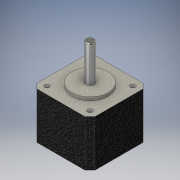
# Autodesk Inventor part: 14HM11
Saved by Autodesk Inventor 2019 (Build 230136000, 136)
## iProperties
Created: 2018-10-31
Part Number: 14HM11
Material: Generic
Document SubType Name: Modeling
Designer: Billy
Density: 3.38062 g/cm^3
Appearance: Default
Mass: 120 g
Surface Area: 68.6294 cm^2
Volume: 35.4965 cm^3
Author: Billy
Autodesk Inventor part; units mm, degrees
ref_plane "YZ Plane" through (0, 0, 0) normal (1, 0, 0) x (0, 1, 0)
ref_plane "XZ Plane" through (0, 0, 0) normal (0, 1, 0) x (-1, 0, 0)
ref_plane "XY Plane" through (0, 0, 0) normal (0, 0, 1) x (1, 0, 0)
sketch "Sketch1" plane through (0, 0, 0) normal (0, 1, 0) x (-1, 0, 0)
  line L0 (-17.6, 0) -> (-17.6, -17.6)
  line L1 (-17.6, -17.6) -> (0, -17.6)
  line L2 (17.6, 0) -> (17.6, -17.6)
  line L3 (17.6, -17.6) -> (0, -17.6)
  line L4 (-17.6, 0) -> (-17.6, 17.6)
  line L5 (-17.6, 17.6) -> (0, 17.6)
  line L6 (17.6, 17.6) -> (0, 17.6)
  line L7 (17.6, 0) -> (17.6, 17.6)
  point P0 (0, 0)
  dimension "d0" = 17.6
  dimension "d1" = 17.6
  constraints: 16 end point
  measures "d0" distance of L1.end L0.end
  measures "d1" distance of L0.end L0.start
extrude "Extrusion1" add sketch "Sketch1" along normal blind 28.2
sketch "Sketch2" plane through (0, 28.2, 0) normal (0, 1, 0) x (1, 0, 0)
  circle A0 centre (13, 13) radius 1.5
  circle A1 centre (-13, 13) radius 1.5
  circle A2 centre (13, -13) radius 1.5
  circle A3 centre (-13, -13) radius 1.5
  point P0 (0, 0)
  dimension "d4" = 3
  dimension "d5" = 3
  dimension "d6" = 3
  dimension "d7" = 3
  constraints: 4 centre point
  measures "d4" diameter of A0
  measures "d5" diameter of A1
  measures "d6" diameter of A2
  measures "d7" diameter of A3
extrude "Extrusion2" cut sketch "Sketch2" against normal blind 4.5
chamfer "Chamfer1" distance 3 angle 45 4 edges at (17.6, 14.1, 17.6) (17.6, 14.1, -17.6) (-17.6, 14.1, 17.6) (-17.6, 14.1, -17.6)
sketch "Sketch3" plane through (0, 28.2, 0) normal (0, 1, 0) x (1, 0, 0)
  circle A0 centre (0, 0) radius 11
  dimension "d13" = 22
  constraints: 1 centre point, 1 coincident
  measures "d13" diameter of A0
extrude "Extrusion3" add sketch "Sketch3" along normal blind 2
sketch "Sketch4" plane through (0, 30.2, 0) normal (0, 1, 0) x (1, 0, 0)
  circle A0 centre (0, 0) radius 2.5
  dimension "d16" = 5
  constraints: 1 centre point, 1 coincident
  measures "d16" diameter of A0
extrude "Extrusion4" add sketch "Sketch4" along normal blind 22
chamfer "Chamfer2" distance 0.5 angle 45 1 edges at (-2.5, 52.2, 0)
body "Solid1"
